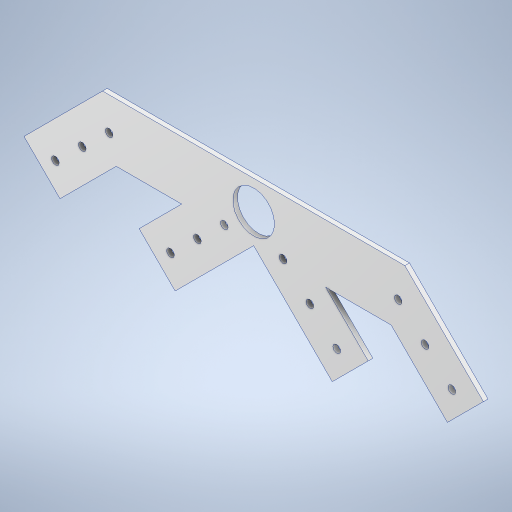
# Autodesk Inventor part: CH1-01-KneePivotPlate
Saved by Autodesk Inventor 2023 (Build 270158000, 158)
## iProperties
Created: 2023-03-03
Part Number: CH1-01-KneePivotPlate
Material: Aluminum 6061
Document SubType Name: Modeling
Designer: megan
Density: 2.7 g/cm^3
Appearance: Aluminum - Flat
Mass: 134.421 g
Surface Area: 352.442 cm^2
Volume: 49.7856 cm^3
Author: megan
Autodesk Inventor part; units mm, degrees
ref_plane "YZ Plane" through (0, 0, 0) normal (1, 0, 0) x (0, 1, 0)
ref_plane "XZ Plane" through (0, 0, 0) normal (0, 1, 0) x (-1, 0, 0)
ref_plane "XY Plane" through (0, 0, 0) normal (0, 0, 1) x (1, 0, 0)
sketch "Sketch1" plane through (0, 0, 0) normal (0, 0, 1) x (1, 0, 0)
  circle A0 centre (0, 0) radius 14.31
  line L0 (-78.5772, -49.1858) -> (-49.3914, -20)
  line L1 (0, -92.6578) -> (0, 38.7763) projected
  line L2 (0, -20) -> (-53.8815, -73.8815)
  line L3 (-53.8815, -73.8815) -> (-78.5772, -49.1858)
  line L4 (0, 20) -> (-103.6841, 20)
  line L5 (-103.6841, 20) -> (-157.5656, -33.8815)
  line L6 (-157.5656, -33.8815) -> (-132.8699, -58.5772)
  line L7 (-132.8699, -58.5772) -> (-94.2927, -20)
  line L8 (-94.2927, -20) -> (-49.3914, -20)
  line L9 (78.5772, -49.1858) -> (49.3914, -20)
  line L10 (0, -20) -> (53.8815, -73.8815)
  line L11 (53.8815, -73.8815) -> (78.5772, -49.1858)
  line L12 (0, 20) -> (103.6841, 20)
  line L13 (103.6841, 20) -> (157.5656, -33.8815)
  line L14 (157.5656, -33.8815) -> (132.8699, -58.5772)
  line L15 (132.8699, -58.5772) -> (94.2927, -20)
  line L16 (94.2927, -20) -> (49.3914, -20)
  line L17 (0, -20) -> (-10.1971, -30.1971)
  point P0 (-68.6659, -39.2745)
  dimension "d1" = 28.62
  dimension "d4" = 76.2
  dimension "d6" = 45
  dimension "d15" = 34.925
  dimension "d59" = 34.925
  dimension "d61" = 101.6
  dimension "d62" = 40
  dimension "d63" = 20
  constraints: 34 end point, 7 symmetric about line, 4 parallel, 4 point on line, 3 perpendicular, 1 centre point, 1 horizontal
  measures "d1" diameter of A0
  measures "d4" distance of L2.start L2.end
  measures "d6" angle of L2 L1
  measures "d15" distance between parallel lines of L2 L0
  measures "d59" distance of L5.end L6.end
  measures "d61" distance between parallel lines of L2 L5
  measures "d62" distance between parallel lines of L8 L4
  measures "d63" distance of point (0, 0) L2.start
extrude "Extrusion1" add sketch "Sketch1" along normal blind 3.175 contours A0 L1 L12 L13 L14 L15 L16 L9 L11 L10 | A0 L1 L2 L3 L0 L8 L7 L6 L5 L4
sketch "Sketch3" plane through (0, 0, 3.175) normal (0, 0, 1) x (1, 0, 0)
  line L0 (53.8815, -73.8815) -> (78.5772, -49.1858) projected
  line L1 (78.5772, -49.1858) -> (49.3914, -20) projected
  line L2 (49.3914, -20) -> (94.2927, -20) projected
  line L3 (94.2927, -20) -> (132.8699, -58.5772) projected
  line L4 (132.8699, -58.5772) -> (157.5656, -33.8815) projected
  line L5 (157.5656, -33.8815) -> (103.6841, 20) projected
  line L6 (103.6841, 20) -> (-103.6841, 20) projected
  line L7 (-103.6841, 20) -> (-157.5656, -33.8815) projected
  line L8 (-157.5656, -33.8815) -> (-132.8699, -58.5772) projected
  line L9 (-132.8699, -58.5772) -> (-94.2927, -20) projected
  line L10 (-94.2927, -20) -> (-49.3914, -20) projected
  line L11 (-49.3914, -20) -> (-78.5772, -49.1858) projected
  line L12 (-78.5772, -49.1858) -> (-53.8815, -73.8815) projected
  line L13 (-53.8815, -73.8815) -> (0, -20) projected
  line L14 (0, -20) -> (53.8815, -73.8815) projected
  circle A0 centre (0, 0) radius 14.31 projected
  line L15 (-145.2178, -46.2294) -> (-75.3998, 20)
  line L16 (-66.2294, -61.5337) -> (19.7221, 20)
  circle A1 centre (-136.0007, -37.486) radius 2.65
  circle A2 centre (-117.5728, -20.0053) radius 2.65
  circle A3 centre (-99.1449, -2.5246) radius 2.65
  circle A4 centre (-57.0123, -52.7903) radius 2.65
  circle A5 centre (-38.5844, -35.3096) radius 2.65
  circle A6 centre (-20.1566, -17.8289) radius 2.65
  dimension "d64" = 5.3
  dimension "d67" = 25.4
  dimension "d72" = 12.7
  dimension "d73" = 12.7
  dimension "d76" = 25.4
  constraints: 6 centre point, 4 end point, 4 point on line, 2 midpoint, 1 equal radius, 1 parallel, 10 other
  measures "d64" diameter of A1
  measures "d67" distance of A1.centre A2.centre
  measures "d72" distance from line of L8 A1.centre
  measures "d73" distance from line of L12 A4.centre
  measures "d76" distance of A4.centre A5.centre
extrude "Extrusion3" cut sketch "Sketch3" against normal blind 25.4 contours A4 L16 | L16 A4 | A5 L16 | L16 A5 | A6 L16 | L16 A6 | A3 L15 | L15 A3 | A1 L15 | L15 A1 | A2 L15 | L15 A2
mirror "Mirror2" about plane through (0, 0, 0) normal (1, 0, 0) of "Extrusion3"
equation "\"d1\" = bearingDiameter"
equation "\"d4\" = boltedLength"
equation "\"d6\" = 0.5 * theta12"
equation "\"d59\" = d15"
equation "\"d61\" = gearboxLength"
equation "\"d62\" = plateHeight"
equation "\"d63\" = 0.5 * plateHeight"
equation "\"topDiameter\" = 45"
equation "\"bearingDiameter\" = 28.62"
equation "\"plateThickness\" = 6.35"
equation "\"theta12\" = 90deg"
equation "\"gearboxLength\" = 101.6"
equation "\"boltedLength\" = 76.2"
equation "\"topDiameter_1\" = 25"
equation "\"shaftLength_1\" = 76.2"
equation "\"bearingDiameter_1\" = 28.62"
equation "\"plateThickness_1\" = 6.35"
equation "\"theta12_1\" = 100deg"
equation "\"boltDiameter_1\" = 6"
equation "\"gearboxLength_1\" = 101.6"
equation "\"boltedLength_1\" = 76.2"
equation "\"innerBoltSpacing_1\" = 12.7"
equation "\"outerBoltSpacing_1\" = 12.7"
equation "\"shaftLength\" = 76.2"
equation "\"boltDiameter\" = 5.3"
equation "\"outerBoltSpacing\" = 12.7"
equation "\"innerBoltSpacing\" = 12.7"
equation "\"plateHeight\" = 40"
body "Solid1"
